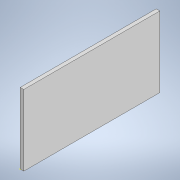
# Autodesk Inventor part: goradol
Saved by Autodesk Inventor 2020 (Build 240168000, 168)
## iProperties
Created: 2020-03-28
Part Number: goradol
Material: Ogólny
Document SubType Name: Modeling
Designer: niedz
Density: 1 g/cm^3
Appearance: Domyślna
Author: niedz
Autodesk Inventor part; units mm, degrees
ref_plane "YZ Plane" through (0, 0, 0) normal (1, 0, 0) x (0, 1, 0)
ref_plane "XZ Plane" through (0, 0, 0) normal (0, 1, 0) x (-1, 0, 0)
ref_plane "XY Plane" through (0, 0, 0) normal (0, 0, 1) x (1, 0, 0)
sketch "Szkic1" plane through (0, 0, 0) normal (1, 0, 0) x (0, 1, 0)
  point P0 (0, 0)
sketch "Szkic2" plane through (0, 0, 0) normal (1, 0, 0) x (0, 1, 0)
  line L0 (0, 0) -> (0, -300)
  line L1 (0, -300) -> (156, -300)
  line L2 (156, -300) -> (156, 0)
  line L3 (156, 0) -> (0, 0)
  dimension "d0" = 300
  dimension "d1" = 156
  dimension "d2" = 300
  constraints: 8 end point, 2 perpendicular, 1 vertical
  measures "d0" distance of L0.start L0.end
  measures "d1" distance of L0.end L1.end
  measures "d2" distance of L1.end L2.end
extrude "Wyciągnięcie proste1" add sketch "Szkic2" along normal blind 8
